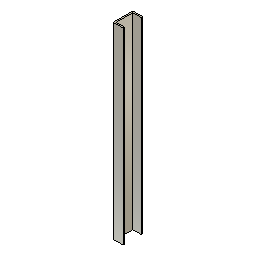
Steel Standing Bracket v6 (Autodesk Fusion 360 design; units mm, degrees)
Autodesk Fusion 360 part; units mm, degrees
sketch "Sketch1" plane through (0, 0, 0) normal (0, 0, 1) x (1, 0, 0)
  line L0 (0, 0) -> (21.0566, 0)
  line L1 (21.0566, 0) -> (21.0566, 41.3258)
  line L2 (21.0566, 41.3258) -> (0, 41.3258)
  line L3 (0, 41.3258) -> (0, 0)
  line L4 (0, 20.6629) -> (21.0566, 20.6629) construction
  line L5 (0, 38.1508) -> (21.0566, 38.1508)
  line L6 (21.0566, 38.1508) -> (21.0566, 3.175) construction
  line L7 (21.0566, 3.175) -> (0, 3.175)
  line L8 (0, 3.175) -> (0, 38.1508) construction
  line L9 (0, 38.1508) -> (21.0566, 3.175) construction
  line L10 (21.0566, 38.1508) -> (0, 3.175) construction
  line L11 (3.175, 38.1508) -> (3.175, 3.175)
  point P0 (10.5283, 20.6629)
  point P1 (0, 20.6629)
  dimension "d1" = 41.3258
  dimension "d2" = 21.0566
  dimension "d3" = 3.175
  dimension "d4" = 3.175
  constraint horizontal L0
  constraint vertical L1
  constraint horizontal L2
  constraint vertical L3
  constraint coincident L0.start L3.end
  constraint midpoint L3 P1
  constraint midpoint L1 L4.end
  constraint horizontal L5
  constraint perpendicular L5 L6
  constraint parallel L5 L7
  constraint parallel L6 L8
  constraint coincident L9 P0
  constraint coincident L10 P0
  constraint coincident L3 L5.start
  constraint midpoint L4 P0
  constraint coincident L5 L11.start
  constraint coincident L7 L11.end
  constraint perpendicular L7 L11
  constraint coincident P1 L4.start
  measures "d1" distance of L0.start L2.end
  measures "d2" distance of L1.end L2.end
  measures "d3" distance of L3 L11
  measures "d4" distance of L2 L5
extrude "Extrude1" add sketch "Sketch1" along normal blind 395 contours L0 L1 L3 L7 | L3 L5 L7 L11 | L1 L2 L3 L5
sketch "Sketch2" plane through (0, 0, 395) normal (0, 0, 1) x (-1, 0, 0)
  line L0 (-21.0566, -38.1508) -> (-21.0566, -41.3258)
  line L1 (-21.0566, -41.3258) -> (0, -41.3258)
  line L2 (0, -41.3258) -> (0, 0)
  line L3 (0, 0) -> (-21.0566, 0)
  line L4 (-21.0566, 0) -> (-21.0566, -3.175)
  line L5 (-21.0566, -3.175) -> (-3.175, -3.175)
  line L6 (-3.175, -3.175) -> (-3.175, -38.1508)
  line L7 (-3.175, -38.1508) -> (-21.0566, -38.1508)
  point P0 (0, -20.6629)
